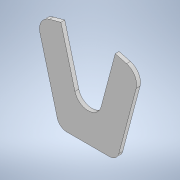
# Autodesk Inventor part: V-slidePlate
Saved by Autodesk Inventor 2022.2 (Build 262287030, 287C)
## iProperties
Created: 2023-04-14
Part Number: V-slidePlate
Material: Generic
Document SubType Name: Modeling
Designer: jak27277
Density: 1 g/cm^3
Appearance: Default
Author: jak27277
Autodesk Inventor part; units mm, degrees
ref_plane "YZ Plane" through (0, 0, 0) normal (1, 0, 0) x (0, 1, 0)
ref_plane "XZ Plane" through (0, 0, 0) normal (0, 1, 0) x (-1, 0, 0)
ref_plane "XY Plane" through (0, 0, 0) normal (0, 0, 1) x (1, 0, 0)
sketch "Sketch1" plane through (0, 0, 0) normal (0, 0, 1) x (1, 0, 0)
  line L0 (0, 0) -> (0, 199.3889) construction
  line L1 (-21.4783, 64.1374) -> (-44.4526, 150.5169)
  line L2 (-44.4526, 150.5169) -> (-62.8626, 145.6204)
  line L3 (-78.6283, 118.4295) -> (-50.2666, 11.7946)
  line L4 (-34.925, 0) -> (0, 0)
  line L5 (21.4783, 64.1374) -> (44.4526, 150.5169)
  line L6 (44.4526, 150.5169) -> (62.8626, 145.6204)
  line L7 (78.6283, 118.4295) -> (50.2666, 11.7946)
  line L8 (34.925, 0) -> (0, 0)
  arc A0 (-21.4783, 64.1374) -> (21.4783, 64.1374) centre (0, 69.85) ccw
  arc A1 (-62.8626, 145.6204) -> (-78.6283, 118.4295) centre (-57.15, 124.1421) ccw
  arc A2 (78.6283, 118.4295) -> (62.8626, 145.6204) centre (57.15, 124.1421) ccw
  arc A3 (-50.2666, 11.7946) -> (-34.925, 0) centre (-34.925, 15.875) ccw
  arc A4 (34.925, 0) -> (50.2666, 11.7946) centre (34.925, 15.875) ccw
  point P0 (-84.3409, 139.9078)
  point P1 (-47.1296, 0)
  point P2 (84.3409, 139.9078)
  point P3 (47.1296, 0)
  dimension "d0" = 69.85
  dimension "d1" = 22.225
  dimension "d2" = 15.875
  dimension "d3" = 34.925
  dimension "d4" = 41.275
  dimension "d5" = 57.15
  dimension "d6" = 22.225
  constraints: 18 end point, 10 point on circle, 9 tangent, 8 point on line, 5 centre point, 4 symmetric about line, 2 equal radius, 1 horizontal, 1 parallel, 1 perpendicular, 1 vertical
  measures "d0" distance from line of L8 A0.centre
  measures "d1" radius of A1
  measures "d2" radius of A3
  measures "d3" distance of L8.start L0.start
  measures "d4" distance between parallel lines of L7 L5
  measures "d5" horizontal distance of A2.centre A0.centre
  measures "d6" radius of A0
extrude "Extrusion1" add sketch "Sketch1" along normal blind 6.35
body "Solid1"
